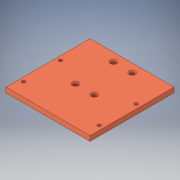
# Autodesk Inventor part: BatteryTop
Saved by Autodesk Inventor 2019 (Build 230136000, 136)
## iProperties
Created: 2018-12-22
Part Number: BatteryTop
Material: Generic
Document SubType Name: Modeling
Designer: james
Density: 1 g/cm^3
Appearance: Default(1)
Author: james
Autodesk Inventor part; units mm, degrees
ref_plane "YZ Plane" through (0, 0, 0) normal (1, 0, 0) x (0, 1, 0)
ref_plane "XZ Plane" through (0, 0, 0) normal (0, 1, 0) x (-1, 0, 0)
ref_plane "XY Plane" through (0, 0, 0) normal (0, 0, 1) x (1, 0, 0)
sketch "Sketch1" plane through (0, 0, 0) normal (0, 1, 0) x (-1, 0, 0)
  line L0 (23.6643, 73.3874) -> (-103.3357, 73.3874)
  line L1 (-103.3357, 73.3874) -> (-103.3357, -53.6126)
  line L2 (-103.3357, -53.6126) -> (23.6643, -53.6126)
  line L3 (23.6643, -53.6126) -> (23.6643, 73.3874)
  point P0 (0, 0)
  dimension "d0" = 127
  dimension "d1" = 127
  constraints: 8 end point, 2 parallel, 1 horizontal, 1 perpendicular
  measures "d0" distance of L2.end L0.start
  measures "d1" distance of L0.start L0.end
extrude "Extrusion1" add sketch "Sketch1" along normal blind 7.62
sketch "Sketch2" plane through (0, 7.62, 0) normal (0, 1, 0) x (1, 0, 0)
  line L0 (-23.6643, 53.6126) -> (-23.6643, -73.3874) projected
  line L1 (103.3357, 53.6126) -> (-23.6643, 53.6126) projected
  line L2 (103.3357, -73.3874) -> (103.3357, 53.6126) projected
  point P0 (0, 0)
  point P1 (-17.3143, -53.0674)
  point P2 (-17.3143, 2.8126)
  point P3 (96.9857, -53.0674)
  point P4 (96.9857, 2.8126)
  dimension "d4" = 0
  dimension "d5" = 6.35
  dimension "d6" = 50.8
  dimension "d7" = 55.88
  dimension "d8" = 0
  dimension "d9" = 0
  dimension "d10" = 0
  dimension "d11" = 6.35
  measures "d4" horizontal distance of point (-17.314, -53.067) point (-17.314, 2.813)
  measures "d5" distance from line of L0 point (-17.314, -53.067)
  measures "d6" distance from line of L1 point (-17.314, 2.813)
  measures "d7" distance of point (-17.314, -53.067) point (-17.314, 2.813)
  measures "d8" vertical distance of point (96.986, 2.813) point (-17.314, 2.813)
  measures "d9" vertical distance of point (-17.314, -53.067) point (96.986, -53.067)
  measures "d10" horizontal distance of point (96.986, 2.813) point (96.986, -53.067)
  measures "d11" distance from line of L2 point (96.986, -53.067)
hole "Hole1" at (-17.3143, 7.62, 53.0674) at (-17.3143, 7.62, -2.8126) at (96.9857, 7.62, 53.0674) at (96.9857, 7.62, -2.8126) direction (0, -1, 0) diameter 5.08 end through all
sketch "Sketch3" plane through (0, 7.62, 0) normal (0, 1, 0) x (1, 0, 0)
  line L0 (103.3357, 53.6126) -> (-23.6643, 53.6126) projected
  line L1 (-23.6643, 53.6126) -> (-23.6643, -73.3874) projected
  line L2 (103.3357, -73.3874) -> (103.3357, 53.6126) projected
  point P0 (0, 0)
  point P1 (24.5957, 40.9126)
  point P2 (52.9421, 40.9126)
  point P3 (24.5957, -16.4406)
  point P4 (52.9421, -16.4406)
  dimension "d19" = 28.3464
  dimension "d20" = 0
  dimension "d21" = 57.3532
  dimension "d22" = 0
  dimension "d23" = 0
  dimension "d24" = 0
  dimension "d25" = 12.7
  dimension "d26" = 48.26
  dimension "d27" = 50.3936
  measures "d19" distance of point (52.942, 40.913) point (24.596, 40.913)
  measures "d20" vertical distance of point (24.596, 40.913) point (52.942, 40.913)
  measures "d21" distance of point (24.596, -16.441) point (24.596, 40.913)
  measures "d22" horizontal distance of point (24.596, 40.913) point (24.596, -16.441)
  measures "d23" horizontal distance of point (52.942, -16.441) point (52.942, 40.913)
  measures "d24" vertical distance of point (52.942, -16.441) point (24.596, -16.441)
  measures "d25" distance from line of L0 point (24.596, 40.913)
  measures "d26" distance from line of L1 point (24.596, 40.913)
  measures "d27" distance from line of L2 point (52.942, 40.913)
hole "Hole2" at (24.5957, 7.62, -40.9126) at (52.9421, 7.62, -40.9126) at (24.5957, 7.62, 16.4406) at (52.9421, 7.62, 16.4406) direction (0, -1, 0) diameter 6.35 end through all countersink diameter 9.525 countersink angle 82
body "Solid1"
